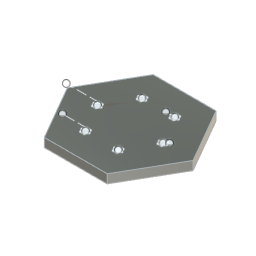
NixOS Logo ShelfMount (Autodesk Fusion 360 design; units mm, degrees)
Autodesk Fusion 360 part; units mm, degrees
sketch "Sketch1" plane through (0, 0, 0) normal (0, 0, 1) x (1, 0, 0)
  line L0 (3.1266, 0.0539) -> (-21.8734, -43.2474)
  line L1 (-21.8734, -43.2474) -> (3.1266, -86.5486)
  line L2 (3.1266, -86.5486) -> (53.1266, -86.5486)
  line L3 (53.1266, -86.5486) -> (78.1266, -43.2474)
  line L4 (78.1266, -43.2474) -> (53.1266, 0.0539)
  line L5 (53.1266, 0.0539) -> (3.1266, 0.0539)
  point P0 (28.1266, -43.2474)
  dimension "d1" = 50
  measures "d1" distance of L0.start L4.end
extrude "Extrude1" add sketch "Sketch1" along normal blind 7
sketch "Sketch2" plane through (0, 0, 7) normal (0, 0, 1) x (-1, 0, 0)
  line L0 (-53.1266, -0.0539) -> (-3.1266, -0.0539)
  line L1 (-3.1266, -0.0539) -> (21.8734, 43.2474)
  line L2 (21.8734, 43.2474) -> (-3.1266, 86.5486)
  line L3 (-3.1266, 86.5486) -> (-53.1266, 86.5486)
  line L4 (-53.1266, 86.5486) -> (-78.1266, 43.2474)
  line L5 (-78.1266, 43.2474) -> (-53.1266, -0.0539)
  line L6 (-13.626, 18.1326) -> (-12.126, 20.7307)
  line L7 (-12.126, 20.7307) -> (-13.626, 23.3288)
  line L8 (-13.626, 23.3288) -> (-16.626, 23.3288)
  line L9 (-16.626, 23.3288) -> (-18.126, 20.7307)
  line L10 (-18.126, 20.7307) -> (-16.626, 18.1326)
  line L11 (-16.626, 18.1326) -> (-13.626, 18.1326)
  line L12 (-44.126, 20.7307) -> (-42.626, 18.1326)
  line L13 (-42.626, 18.1326) -> (-39.626, 18.1326)
  line L14 (-39.626, 18.1326) -> (-38.126, 20.7307)
  line L15 (-38.126, 20.7307) -> (-39.626, 23.3288)
  line L16 (-39.626, 23.3288) -> (-42.626, 23.3288)
  line L17 (-42.626, 23.3288) -> (-44.126, 20.7307)
  line L18 (-44.126, 20.7307) -> (-33.8895, 20.7307) construction
  line L19 (-55.626, 40.6493) -> (-52.626, 40.6493)
  line L20 (-52.626, 40.6493) -> (-51.126, 43.2473)
  line L21 (-51.126, 43.2473) -> (-52.626, 45.8454)
  line L22 (-52.626, 45.8454) -> (-55.626, 45.8454)
  line L23 (-55.626, 45.8454) -> (-57.126, 43.2473)
  line L24 (-57.126, 43.2473) -> (-55.626, 40.6493)
  line L25 (-55.626, 40.6493) -> (-56.8973, 40.6493) construction
  line L26 (-38.126, 65.764) -> (-39.626, 68.3621)
  line L27 (-39.626, 68.3621) -> (-42.626, 68.3621)
  line L28 (-42.626, 68.3621) -> (-44.126, 65.764)
  line L29 (-44.126, 65.764) -> (-42.626, 63.1659)
  line L30 (-42.626, 63.1659) -> (-39.626, 63.1659)
  line L31 (-39.626, 63.1659) -> (-38.126, 65.764)
  line L32 (-38.126, 65.764) -> (-41.1962, 65.764) construction
  line L33 (-13.626, 63.1659) -> (-12.126, 65.764)
  line L34 (-12.126, 65.764) -> (-13.626, 68.3621)
  line L35 (-13.626, 68.3621) -> (-16.626, 68.3621)
  line L36 (-16.626, 68.3621) -> (-18.126, 65.764)
  line L37 (-18.126, 65.764) -> (-16.626, 63.1659)
  line L38 (-16.626, 63.1659) -> (-13.626, 63.1659)
  line L39 (-13.626, 63.1659) -> (5.8693, 63.1659) construction
  line L40 (-0.626, 40.6493) -> (0.874, 43.2473)
  line L41 (0.874, 43.2473) -> (-0.626, 45.8454)
  line L42 (-0.626, 45.8454) -> (-3.626, 45.8454)
  line L43 (-3.626, 45.8454) -> (-5.126, 43.2473)
  line L44 (-5.126, 43.2473) -> (-3.626, 40.6493)
  line L45 (-3.626, 40.6493) -> (-0.626, 40.6493)
  line L46 (-0.626, 40.6493) -> (25.3601, 40.6493) construction
  point P0 (-15.126, 20.7307)
  point P1 (-41.126, 20.7307)
  point P2 (-54.126, 43.2473)
  point P3 (-41.126, 65.764)
  point P4 (-15.126, 65.764)
  point P5 (-2.126, 43.2473)
  dimension "d4" = 3
  dimension "d5" = 60
  dimension "d6" = 3
  dimension "d7" = 60
  dimension "d8" = 3
  dimension "d9" = 60
  dimension "d10" = 3
  dimension "d11" = 60
  dimension "d12" = 3
  dimension "d13" = 60
  dimension "d15" = 20
  dimension "d16" = 20
  dimension "d17" = 20
  dimension "d20" = 3
  dimension "d21" = 20
  dimension "d22" = 20
  dimension "d23" = 20
  dimension "d26" = 18.1865
  dimension "d27" = 18.1866
  dimension "d28" = 18.187
  dimension "d29" = 18.187
  constraint horizontal L18
  constraint horizontal L25
  constraint horizontal L32
  constraint horizontal L39
  constraint horizontal L46
  constraint parallel L0 L11
  constraint collinear L11 L13
  constraint collinear L12 L24
  constraint collinear L23 L28
  constraint collinear L27 L35
  measures "d4" distance of L12.start L12.end
  measures "d5" angle of L12 L18
  measures "d6" distance of L19.start L23.end
  measures "d7" angle of L24 L25
  measures "d8" distance of L26.start L30.end
  measures "d9" angle of L31 L32
  measures "d10" distance of L33.start L33.end
  measures "d11" angle of L33 L39
  measures "d12" distance of L40.start L40.end
  measures "d13" angle of L40 L46
  measures "d15" distance of L16.end L19.end
  measures "d16" distance of L21.end L29.end
  measures "d17" distance of L26.start L36.end
  measures "d20" horizontal distance of L6.start L10.end
  measures "d21" distance of L9.end L14.end
  measures "d22" distance of L7.end L44.end
  measures "d23" distance of L33.start L42.end
  measures "d26" distance of L0 L11
  measures "d27" distance of L3 L35
  measures "d28" distance of L5 L12
  measures "d29" distance of L4 L23
extrude "Extrude2" cut sketch "Sketch2" against normal blind 5.2 contours L6 L7 L8 L9 L10 L11 | L12 L13 L14 L15 L16 L17 | L19 L20 L21 L22 L23 L24 | L26 L27 L28 L29 L30 L31 | L33 L34 L35 L36 L37 L38 | L40 L41 L42 L43 L44 L45
sketch "Sketch4" plane through (0, 0, 0) normal (0, 0, -1) x (1, 0, 0)
  line L0 (3.1266, -0.0539) -> (53.1266, -0.0539)
  line L1 (53.1266, -0.0539) -> (78.1266, 43.2474)
  line L2 (78.1266, 43.2474) -> (53.1266, 86.5486)
  line L3 (53.1266, 86.5486) -> (3.1266, 86.5486)
  line L4 (3.1266, 86.5486) -> (-21.8734, 43.2474)
  line L5 (-21.8734, 43.2474) -> (3.1266, -0.0539)
  circle A0 centre (28.127, 43.2471) radius 3
  dimension "d38" = 6
  dimension "d39" = 43.3015
  dimension "d40" = 43.3015
  dimension "d41" = 43.3008
  measures "d38" diameter of A0
  measures "d39" distance of L3 A0.centre
  measures "d40" distance of L5 A0.centre
  measures "d41" distance of L1 A0.centre
extrude "Extrude4" cut sketch "Sketch4" against normal blind 4 contours A0
fillet "Fillet1" radius 1 1 edges at (25.33, -44.332, 0)
